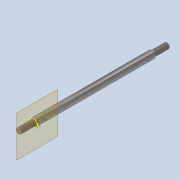
# Autodesk Inventor part: GearShaft_1
Saved by Autodesk Inventor 2021.2 (Build 252289000, 289)
## iProperties
Created: 2020-05-27
Part Number: GearShaft_1
Material: 鉄、鋳鉄
Document SubType Name: Modeling
Designer: Hagihara Yuya
Density: 7.15 g/cm^3
Appearance: 鋼 - つや出し
Mass: 7.01426 g
Surface Area: 10.6434 cm^2
Volume: 0.981016 cm^3
Author: Hagihara Yuya
Autodesk Inventor part; units mm, degrees
ref_plane "YZ Plane" through (0, 0, 0) normal (1, 0, 0) x (0, 1, 0)
ref_plane "XZ Plane" through (0, 0, 0) normal (0, 1, 0) x (-1, 0, 0)
ref_plane "XY Plane" through (0, 0, 0) normal (0, 0, 1) x (1, 0, 0)
sketch "スケッチ1" plane through (0, 0, 0) normal (1, 0, 0) x (0, 1, 0)
  circle A0 centre (0, 0) radius 2
  dimension "d0" = 4
  constraints: 1 centre point, 1 coincident
  measures "d0" diameter of A0
extrude "押し出し1" add sketch "スケッチ1" along normal blind 64
sketch "スケッチ4" plane through (0, 0, 0) normal (-1, 0, 0) x (0, 0, 1)
  circle A0 centre (0, 0) radius 1.5
  dimension "d16" = 3
  constraints: 1 centre point, 1 coincident
  measures "d16" diameter of A0
extrude "押し出し2" add sketch "スケッチ4" along normal blind 8
sketch "スケッチ5" plane through (64, 0, 0) normal (1, 0, 0) x (0, 0, -1)
  circle A0 centre (0, 0) radius 1.5
  dimension "d19" = 3
  constraints: 1 centre point, 1 coincident
  measures "d19" diameter of A0
extrude "押し出し3" add sketch "スケッチ5" along normal blind 8
thread "ねじ1" size "M3x0.5" class "6g" standard "ISO Metric profile" length 8
thread "ねじ2" size "M3x0.5" class "6g" standard "ISO Metric profile" length 8
sketch "スケッチ2" plane through (64, 0, 0) normal (1, 0, 0) x (0, 0, -1)
  circle A0 centre (0, 0) radius 2 projected
  line L0 (0, -2.8) -> (0, 2.8) projected
  point P0 (0, 2)
  constraints: 1 point on line, 1 vertical alignment, 1 other
ref_plane "作業平面1" through (64, 2, 0) normal (0, 1, 0) x (-1, 0, 0)
sketch "スケッチ3" plane through (64, 2, 0) normal (0, 1, 0) x (-1, 0, 0)
  line L0 (64, 0) -> (0, 0)
  line L1 (0, 2) -> (0, -2) projected
  line L2 (-8, 1.5) -> (-8, -1.5) projected
  line L3 (72, -1.5) -> (72, 1.5) projected
  point P0 (4.5, 0)
  point P1 (59.5, 0)
  dimension "d22" = 12.5
  dimension "d23" = 12.5
  constraints: 2 end point, 2 point on line, 1 horizontal, 1 midpoint
  measures "d22" distance from line of L2 point (4.5, 0)
  measures "d23" distance from line of L3 point (59.5, 0)
hole "穴1" at (59.5, 2, 0) at (4.5, 2, 0) direction (0, -1, 0) diameter 2 end through all
equation "\"d23\" = d22"
